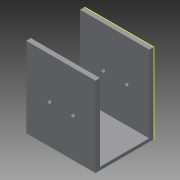
# Autodesk Inventor part: 知能ロボコンギアボックス１
Saved by Autodesk Inventor 2013 (Build 170138000, 138)
## iProperties
Created: 2014-05-31
Part Number: 知能ロボコンギアボックス１
Material: 一般
Document SubType Name: Modeling
Designer: horumo136
Density: 1 g/cm^3
Author: horumo136
Autodesk Inventor part; units mm, degrees
ref_plane "YZ Plane" through (0, 0, 0) normal (1, 0, 0) x (0, 1, 0)
ref_plane "XZ Plane" through (0, 0, 0) normal (0, 1, 0) x (-1, 0, 0)
ref_plane "XY Plane" through (0, 0, 0) normal (0, 0, 1) x (1, 0, 0)
sketch "スケッチ1" plane through (0, 0, 0) normal (0, 1, 0) x (-1, 0, 0)
  line L0 (0, 0) -> (-45, 0)
  line L1 (-45, 0) -> (-45, 2)
  line L2 (-45, 2) -> (0, 2)
  line L3 (0, 2) -> (0, 0)
  dimension "d0" = 45
  dimension "d1" = 2
  constraints: 8 end point, 2 parallel, 1 horizontal, 1 perpendicular
  measures "d0" distance of L1.end L2.end
  measures "d1" distance of L0.end L1.end
extrude "押し出し1" add sketch "スケッチ1" along normal blind 38
sketch "スケッチ2" plane through (0, 0, 2) normal (0, 0, 1) x (1, 0, 0)
  line L0 (45, 0) -> (0, 0) projected
  line L1 (45, 0) -> (45, 38) projected
  line L2 (0, 38) -> (45, 38)
  line L3 (45, 38) -> (45, 35)
  line L4 (45, 35) -> (0, 35)
  line L5 (0, 35) -> (0, 38)
  line L6 (0, 0) -> (45, 0)
  line L7 (45, 0) -> (45, 3)
  line L8 (45, 3) -> (0, 3)
  line L9 (0, 3) -> (0, 0)
  dimension "d4" = 3
  dimension "d5" = 3
  constraints: 16 end point, 4 parallel, 2 horizontal, 2 perpendicular, 2 point on line
  measures "d4" distance of L2.end L3.end
  measures "d5" distance of L7.end L6.end
extrude "押し出し2" add sketch "スケッチ2" along normal blind 50
sketch "スケッチ3" plane through (0, 38, 0) normal (0, 1, 0) x (1, 0, 0)
  line L0 (45, 0) -> (0, 0) projected
  line L1 (0, 0) -> (0, -52) projected
  line L2 (45, -52) -> (0, -52) projected
  line L3 (45, 0) -> (45, -52) projected
sketch "スケッチ4" plane through (0, 0, 0) normal (0, -1, 0) x (1, 0, 0)
  line L0 (0, 0) -> (45, 0) projected
  line L1 (14.737, 0) -> (29.997, 0)
  line L2 (29.997, 0) -> (29.997, 25.5)
  line L3 (29.997, 25.5) -> (14.737, 25.5)
  line L4 (14.737, 25.5) -> (14.737, 0)
  dimension "d8" = 15.26
  dimension "d9" = 25.5
  constraints: 8 end point, 2 parallel, 1 horizontal, 1 perpendicular, 1 point on line
  measures "d8" distance of L3.end L2.end
  measures "d9" distance of L2.end L1.end
hole "穴1" at (14.737, 0, 25.5) at (29.997, 0, 25.5) direction (0, 1, 0) diameter 3 depth 40 tip angle 118
